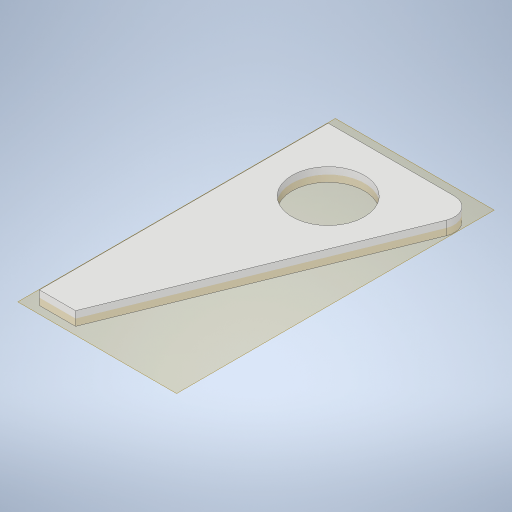
# Autodesk Inventor part: Liftinglug
Saved by Autodesk Inventor 2023 (Build 270158030, 158C)
## iProperties
Created: 2018-09-20
Part Number: Liftinglug
Material: Generic
Document SubType Name: Modeling
Designer: Q
Density: 1 g/cm^3
Appearance: Default(1)
Author: Q
Autodesk Inventor part; units mm, degrees
ref_plane "YZ Plane" through (0, 0, 0) normal (1, 0, 0) x (0, 1, 0)
ref_plane "XZ Plane" through (0, 0, 0) normal (0, 1, 0) x (-1, 0, 0)
ref_plane "XY Plane" through (0, 0, 0) normal (0, 0, 1) x (1, 0, 0)
sketch "Sketch1" plane through (0, 0, 0) normal (0, 1, 0) x (-1, 0, 0)
  line L0 (0, 0) -> (0, 101.6)
  line L1 (0, 101.6) -> (-12.7, 101.6)
  line L2 (0, 0) -> (-44.45, 0)
  line L3 (-12.7, 101.6) -> (-50.3351, 8.735)
  arc A0 (-50.3351, 8.735) -> (-44.45, 0) centre (-44.45, 6.35) ccw
  line L4 (-50.8, 8.1746) -> (-50.8, -12.3493) construction
  circle A1 centre (-22.225, 22.225) radius 12.7
  point P0 (-53.8751, 0)
  dimension "d0" = 101.6
  dimension "d1" = 12.7
  dimension "d4" = 6.35
  dimension "d5" = 50.8
  dimension "d6" = 25.4
  dimension "d7" = 22.225
  dimension "d8" = 22.225
  constraints: 10 end point, 3 tangent, 2 centre point, 2 horizontal, 2 point on circle, 2 point on line, 2 vertical
  measures "d0" distance of L0.start L0.end
  measures "d1" distance of L0.end L1.end
  measures "d4" radius of A0
  measures "d5" distance between parallel lines of L4 L0
  measures "d6" diameter of A1
  measures "d7" distance from line of L0 A1.centre
  measures "d8" distance from line of L2 A1.centre
extrude "Extrusion1" add sketch "Sketch1" along normal blind 4.7625
ref_plane "WP Lug" through (0, 2.3813, 0) normal (0, 1, 0) x (1, 0, 0)
body "Solid1"
